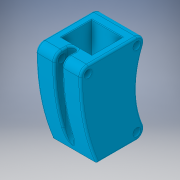
# Autodesk Inventor part: climb slider
Saved by Autodesk Inventor 2017 SP1 (Build 210196100, 196)
## iProperties
Created: 2018-03-18
Part Number: climb slider
Material: ABS Plastic
Document SubType Name: Modeling
Designer: Ben
Density: 1.06 g/cm^3
Appearance: Sky Blue Medium
Mass: 79.7397 g
Surface Area: 252.614 cm^2
Volume: 75.2261 cm^3
Author: Ben
Autodesk Inventor part; units mm, degrees
ref_plane "YZ Plane" through (0, 0, 0) normal (1, 0, 0) x (0, 1, 0)
ref_plane "XZ Plane" through (0, 0, 0) normal (0, 1, 0) x (-1, 0, 0)
ref_plane "XY Plane" through (0, 0, 0) normal (0, 0, 1) x (1, 0, 0)
sketch "Sketch1" plane through (0, 0, 0) normal (0, 1, 0) x (-1, 0, 0)
  line L0 (12.954, 12.954) -> (-12.954, 12.954)
  line L1 (-12.954, 12.954) -> (-12.954, -12.954)
  line L2 (-12.954, -12.954) -> (12.954, -12.954)
  line L3 (12.954, -12.954) -> (12.954, 12.954)
  line L4 (12.954, 12.954) -> (-12.954, -12.954) construction
  line L5 (-12.954, 12.954) -> (12.954, -12.954) construction
  line L6 (19.05, 28.575) -> (-19.05, 28.575)
  line L7 (-19.05, 28.575) -> (-19.05, -25.4)
  line L8 (-19.05, -25.4) -> (19.05, -25.4)
  line L9 (19.05, -25.4) -> (19.05, 28.575)
  line L10 (-12.954, -12.954) -> (-19.05, -12.954) construction
  line L11 (12.954, -12.954) -> (19.05, -12.954) construction
  point P0 (0, 0)
  dimension "d0" = 25.908
  dimension "d48" = 38.1
  dimension "d49" = 28.575
  dimension "d50" = 25.4
  constraints: 24 end point, 4 parallel, 3 perpendicular, 3 point on line, 2 equal length, 2 horizontal, 2 midpoint
  measures "d0" distance of L2.end L1.end
  measures "d48" distance between parallel lines of L9 L7
  measures "d49" distance from line of L6 point (0, 0)
  measures "d50" distance from line of point (0, 0) L8
extrude "Extrusion1" add sketch "Sketch1" along normal blind 76.2
sketch "Sketch2" plane through (19.05, 0, 28.575) normal (1, 0, 0) x (0, 0, -1)
  line L0 (28.575, 0) -> (28.575, 76.2) construction
  line L1 (41.529, 76.2) -> (15.621, 76.2) construction
  line L2 (41.529, 0) -> (41.529, 76.2) construction
  line L3 (15.621, 0) -> (15.621, 76.2) construction
  line L4 (0, 0) -> (53.975, 0) construction
  line L5 (0, 0) -> (0, 76.2) construction
  line L6 (0, 38.1) -> (51.308, 38.1) construction
  circle A0 centre (47.625, 69.85) radius 3.302
  circle A1 centre (47.625, 6.35) radius 3.302
  circle A2 centre (6.35, 69.85) radius 3.302
  line L7 (47.625, 69.85) -> (6.35, 69.85) construction
  arc A3 (53.486538, 67.407692) -> (53.975, 69.85) centre (47.625, 69.85) ccw
  arc A4 (53.975, 6.35) -> (53.486538, 8.792308) centre (47.625, 6.35) ccw
  arc A5 (53.486538, 67.407692) -> (53.486538, 8.792308) centre (123.825, 38.1) ccw
  line L8 (0, 69.85) -> (0, 0)
  line L9 (53.975, 0) -> (0, 0)
  line L10 (0, 0) -> (14.0335, 0)
  line L11 (53.975, 0) -> (53.975, 76.2) construction
  line L12 (47.625, 69.85) -> (47.625, 6.35) construction
  arc A6 (0, 69.85) -> (14.0335, 0) centre (180.851592, 69.85) ccw
  line L13 (53.975, 69.85) -> (53.975, 6.35)
  dimension "d14" = 1.5875
  dimension "d40" = 6.35
  dimension "d45" = 6.35
  dimension "d46" = 6.604
  dimension "d47" = 6.35
  dimension "d51" = 6.35
  constraints: 14 end point, 8 point on circle, 7 centre point, 6 tangent, 5 point on line, 2 coincident, 2 collinear, 2 equal radius, 2 horizontal, 2 midpoint, 1 perpendicular, 1 vertical
  measures "d14" distance from line of L10.end L3
  measures "d40" distance from line of L4 A1.centre
  measures "d45" distance between parallel lines of L7 L1
  measures "d46" diameter of A0
  measures "d47" distance from line of L5 L7.end
  measures "d51" distance between parallel lines of L12 L11
extrude "Extrusion2" cut sketch "Sketch2" against normal through all
chamfer "Chamfer1" distance 0.508 angle 45 8 edges at (12.954, 0, 0) (0, 0, 12.954) (-12.954, 0, 0) (0, 0, -12.954) (-12.954, 76.2, 0) (0, 76.2, -12.954) (12.954, 76.2, 0) (0, 76.2, 12.954)
fillet "Fillet1" radius 6.35 3 edges at (0, 76.2, 28.575) (0, 76.2, -25.4) (0, 0, -25.4)
fillet "Fillet1" radius 0.762 1 edges at (0, 0, 14.5415)
fillet "Fillet2" radius 1.5875 22 edges at (19.05, 74.3402, -23.5402) (19.05, 69.8501, -25.4) (19.05, 68.6047, -25.2767) (19.05, 76.2, 1.5875) (19.05, 69.8501, 28.575) (19.05, 74.3402, 26.7152) (19.05, 0, -2.5082) (19.05, 1.8598, -23.5402) (19.05, 6.3499, -25.4) (19.05, 7.5953, -25.2767) (19.05, 38.1, -19.05) (-19.05, 69.8501, 28.575) (-19.05, 74.3402, 26.7152) (-19.05, 76.2, 1.5875) (-19.05, 68.6047, -25.2767) (-19.05, 69.8501, -25.4) (-19.05, 74.3402, -23.5402) (-19.05, 38.1, -19.05) (-19.05, 1.8598, -23.5402) (-19.05, 6.3499, -25.4) (-19.05, 7.5953, -25.2767) (-19.05, 0, -2.5082)
ref_plane "Work Plane2" through (9.525, 76.2, -19.05) normal (0, 0.9993908, -0.0348995) x (1, 0, 0)
sketch "Sketch6" plane through (9.525, 76.2, -19.05) normal (0, 0.9993908, -0.0348995) x (1, 0, 0)
  line L0 (-9.525, -16.379054) -> (-9.525, -42.635289) construction
  arc A0 (-6.35, -36.411775) -> (-12.7, -36.411775) centre (-9.525, -36.411775) ccw
  line L1 (3.429, -31.966775) -> (-22.479, -31.966775) construction
  line L2 (-6.35, -36.411775) -> (-6.35, -49.111775)
  line L3 (-6.35, -49.111775) -> (-12.7, -49.111775)
  line L4 (-12.7, -49.111775) -> (-12.7, -36.411775)
  arc A1 (-12.7, -36.411775) -> (-6.35, -36.411775) centre (-9.525, -36.411775) ccw construction
  point P0 (-9.525, -33.236775)
  dimension "d53" = 1.27
  dimension "d54" = 3.175
  dimension "d55" = 12.7
  constraints: 8 end point, 5 point on circle, 3 vertical, 2 centre point, 2 point on line, 1 coincident, 1 perpendicular, 1 tangent
  measures "d53" distance from line of L1 point (-9.525, -33.237)
  measures "d54" radius of A0
  measures "d55" distance of L2.start L2.end
extrude "Extrusion5" cut sketch "Sketch6" against normal through all
fillet "Fillet4" radius 1.5875 8 edges at (-0.0327, 5.3481, 16.6814) (-3.175, 41.3197, 26.3104) (-3.175, 74.3402, 26.7152) (-3.175, 76.2, 19.8045) (0, 76.2, 14.207) (3.175, 76.2, 19.8045) (3.175, 74.3402, 26.7152) (3.175, 41.3197, 26.3104)
body "Solid1"
